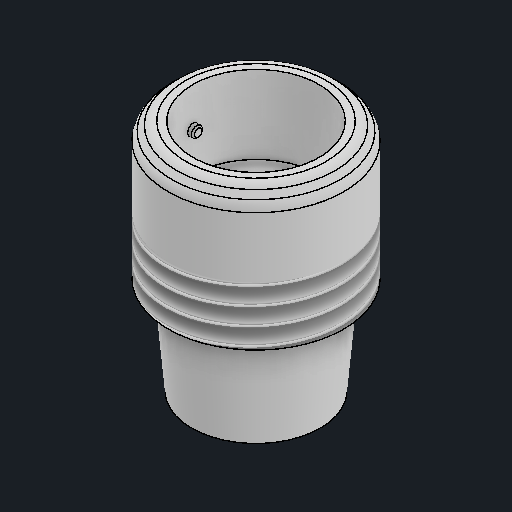
# Autodesk Inventor part: Cyclone Hose Adapter
Saved by Autodesk Inventor 2026.2 (Build 302298000, 298)
## iProperties
Created: 2026-06-17
Part Number: Cyclone Hose Adapter
Material: Generic
Document SubType Name: Modeling
Designer: JoshuaEah
Density: 1 g/cm^3
Appearance: Default
Author: JoshuaEah
Autodesk Inventor part; units mm, degrees
ref_plane "YZ Plane" through (0, 0, 0) normal (1, 0, 0) x (0, 1, 0)
ref_plane "XZ Plane" through (0, 0, 0) normal (0, 1, 0) x (-1, 0, 0)
ref_plane "XY Plane" through (0, 0, 0) normal (0, 0, 1) x (1, 0, 0)
sketch "Sketch1" plane through (0, 0, 0) normal (0, 1, 0) x (-1, 0, 0)
  circle A0 centre (0, 0) radius 16.2
  circle A1 centre (0, 0) radius 22.5
  line L0 (17.6, 1.4) -> (14.8, 1.4)
  line L1 (14.8, 1.4) -> (14.8, -1.4)
  line L2 (14.8, -1.4) -> (17.6, -1.4)
  line L3 (17.6, -1.4) -> (17.6, 1.4)
  line L4 (17.6, 1.4) -> (14.8, -1.4) construction
  line L5 (14.8, 1.4) -> (17.6, -1.4) construction
  line L6 (16.2, 0) -> (14.8, 0)
  line L7 (16.2, 1.4) -> (16.2, -1.4)
  circle A2 centre (0, 0) radius 11
  point P0 (16.1394, -1.4)
  point P1 (16.2, 0)
  dimension "d0" = 32.4
  dimension "d1" = 45
  dimension "d20" = 2.8
  dimension "d21" = 2.8
  dimension "d35" = 22
  constraints: 16 end point, 5 midpoint, 2 centre point, 2 coincident, 2 parallel, 1 horizontal, 1 horizontal alignment, 1 perpendicular, 4 other
  measures "d1" diameter of A1
  measures "d20" distance of L2.end L1.end
  measures "d21" distance of L1.end L0.end
  measures "d35" diameter of A2
extrude "Top" add sketch "Sketch1" along normal blind 10 contours L7 L2 A0 | A0 L0 L7 | L7 L0 L3 L2 | A1
extrude "Middle" add sketch "Sketch1" against normal blind 10 contours L7 L2 A0 | A0 L0 L7 | L7 L0 L3 L2 | A1
extrude "Bottom" add sketch "Sketch1" against normal blind 10 from surface at -10 contours L6 L1 L0 A0 | L7 L2 A0 | A0 L2 L1 L6 | A0 L0 L7 | L7 L0 L3 L2 | L0 L1 L2 A0 | A1
revolve "Cam" add sketch "Sketch1" angle 360 about axis through (-16.2, 0, 0) along (1, 0, 0) contours L7 L2 A0 | A0 L2 L1 L6
chamfer "Cam Chamfer" distance 0.4 angle 45 1 edges at (-14.8, 0, 1.4)
chamfer "Chamfer4" distance 3.175 angle 45 1 edges at (22.5, 10, 0)
fillet "Fillet2" radius 3.175 2 edges at (22.5, 6.825, 0) (19.325, 10, 0)
sketch "Sketch3" plane through (0, -20, 0) normal (0, -1, 0) x (1, 0, 0)
  circle A0 centre (0, 0) radius 22.5 projected
  circle A1 centre (0, 0) radius 16.5
  circle A2 centre (0, 0) radius 11
  circle A3 centre (0, 0) radius 22.5
  dimension "d37" = 33
  dimension "d38" = 22
  dimension "d41" = 45
  constraints: 3 centre point, 3 concentric
  measures "d37" diameter of A1
  measures "d38" diameter of A2
  measures "d41" diameter of A3
extrude "Extrusion6" add sketch "Sketch3" along normal blind 5 contours A0 | A1
extrude "Extrusion7" add sketch "Sketch3" along normal blind 25 from surface at 5 contours A1
draft "FaceDraft1" angle 5 pull direction (0, -1, 0) faces at (16.4465, -41.6667, -1.3277) fixed edges at (-16.5, -50, 0)
thread "Thread2" size "M45x4.5" class "6g" standard "ANSI Metric M Profile" length 15
body "Solid1"
